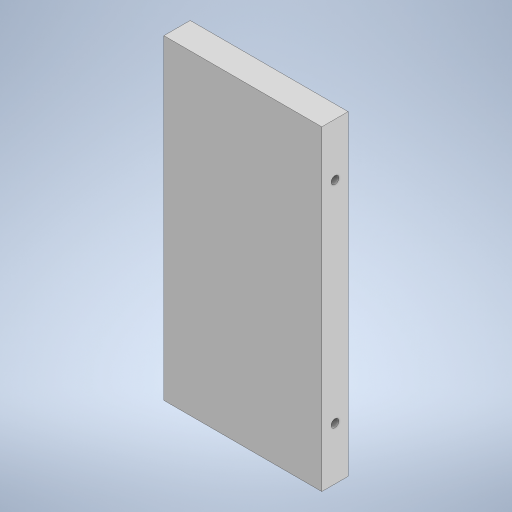
# Autodesk Inventor part: plaque de separation
Saved by Autodesk Inventor 2023 (Build 270158000, 158)
## iProperties
Created: 2022-11-02
Part Number: plaque de separation
Material: Générique
Document SubType Name: Modeling
Designer: Julia
Density: 1 g/cm^3
Appearance: Par défaut
Author: Julia
Autodesk Inventor part; units mm, degrees
ref_plane "YZ Plane" through (0, 0, 0) normal (1, 0, 0) x (0, 1, 0)
ref_plane "XZ Plane" through (0, 0, 0) normal (0, 1, 0) x (-1, 0, 0)
ref_plane "XY Plane" through (0, 0, 0) normal (0, 0, 1) x (1, 0, 0)
sketch "Esquisse1" plane through (0, 0, 0) normal (0, 0, 1) x (1, 0, 0)
  line L0 (22.3904, 80.6375) -> (22.3904, -39.3625)
  line L1 (-37.6096, 80.6375) -> (-37.6096, -39.3625)
  line L2 (-37.6096, -39.3625) -> (22.3904, -39.3625)
  line L3 (-37.6096, 80.6375) -> (22.3904, 80.6375)
  point P0 (0, 0)
  dimension "d0" = 120
  dimension "d1" = 60
  constraints: 8 end point, 2 perpendicular, 2 vertical
  measures "d0" distance of L1.start L1.end
  measures "d1" distance of L1.end L0.end
extrude "Extrusion1" add sketch "Esquisse1" along normal mid plane 10
sketch "Esquisse2" plane through (22.3904, -39.3625, 5) normal (1, 0, 0) x (0, 0, -1)
  circle A0 centre (5, 100) radius 1.5
  line L0 (10, 0) -> (0, 0) projected
  point P0 (5, 39.3625)
  point P1 (5, 0)
  dimension "d10" = 100
  dimension "d11" = 3
  constraints: 1 centre point, 1 midpoint
  measures "d10" distance of point (5, 0) A0.centre
  measures "d11" diameter of A0
sketch "Esquisse3" plane through (22.3904, -39.3625, 5) normal (1, 0, 0) x (0, 0, -1)
  circle A0 centre (5, 20) radius 1.5
  line L0 (10, 0) -> (0, 0) projected
  circle A1 centre (5, 100) radius 1.5
  point P0 (5, 39.3625)
  point P1 (5, 0)
  dimension "d4" = 20
  dimension "d5" = 3
  dimension "d6" = 100
  dimension "d7" = 3
  constraints: 2 centre point, 1 midpoint
  measures "d4" distance of point (5, 0) A0.centre
  measures "d5" diameter of A0
  measures "d6" vertical distance of L0.start A1.centre
  measures "d7" diameter of A1
extrude "Extrusion2" cut sketch "Esquisse3" against normal through all contours A0
extrude "Extrusion3" cut sketch "Esquisse2" against normal blind 60
